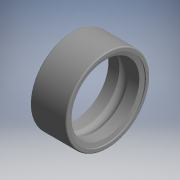
# Autodesk Inventor part: W 638/3-2Z_PART2
Saved by Autodesk Inventor 2017.3 (Build 213256000, 256)
## iProperties
Part Number: W 638/3-2Z_PART2
Material: Generic
Catalog Web Link: www.cadenas.de
Description: -Deep groove ball bearings
Vendor: SKF
Document SubType Name: Modeling
Designer: partserver
Manufacturer: SKF
Mass: 0.0355335 g
Surface Area: 1.47761 cm^2
Volume: 0.0355335 cm^3
Density: 1 g/cm^3
Appearance: PSOLRGB-175-175-175
Category: PARTsolutions
Company: SKF
Title: W 638/3-2Z_PART2
Author: Cadenas PARTsolutions
Comments: Deep groove ball bearings
PSOL_IDENT_0: {$CADENAS_DATA\23d-libs\skf_r32\bearings_units_and_housings\ball_bearings\deep_groove_ball_bearings\
PSOL_IDENT_1: bb1_001_101.prj},199 {VTYP=3D},{NB=W 638/3-2Z_PART2},{LINA=W 638/3-2Z_PART2},{NN=BB1_001_101_PART2},
PSOL_IDENT_2: {NOPRJ=TRUE},{DATE=03.04.2020 14:22:31},{GEOMDATE=30.03.2020 16:10:03},{VERSION=},{LINEID=19220},{WB
PSOL_IDENT_3: VAR=},{WBNUMERIC=}  {NB=W 638/3-2Z_PART2},{LINA=W 638/3-2Z_PART2},{KT=DUMMY},{DESIGNATION=W 638/3-2Z
PSOL_IDENT_4: },{DD=3.000},{D=7.000},{B=3.000},{C=0.000},{DD1=0.00},{DD2=3.90},{D1=0.00},{D2=6.35},{D3=0.000},{D4=
PSOL_IDENT_5: 0.000},{HH=MIN},{BB=0.000},{FF=0.00},{R0MAX=MIN},{R0=MIN},{R12=0.10},{PITCH=5.00},{DW=1.000},{DDAMIN=
PSOL_IDENT_6: 3.700},{DDAMAX=3.800},{DDBMIN=MIN},{DDBMAX=MIN},{DBMIN=MIN},{DAMAX=6.500},{BBAMIN=MIN},{CAMAX=MIN},{
PSOL_IDENT_7: RAMAX=0.100},{LOAD1=0.178},{LOAD2=0.057},{LOAD3=0.002},{SPEED1=160000},{SPEED2=80000},{KR=0.020},{F0=
PSOL_IDENT_8: 7.100},{Z=8},{II=1},{MASS=0.000},{BEARING=W 638/3-2Z},{RING=},{HELP=0.665},{HELP2=0.325},{DD1ALG=2.0
PSOL_IDENT_9: 00},{YALG=2.175},{PITCH1=5.000},{DW1=1.000},{YALG1=2.835},{HALG1=0.665},{SH=1.950},{CU=0.400},{DESIG
PSOL_IDENT_10: N=dgbbw2z},{HALG=0.675},{B1=0},{SHIELDHELP=2}
NB: W 638/3-2Z_PART2
NT: Deep groove ball bearings
NBSYN: $DESIGNATION._PART2
LINA: W 638/3-2Z_PART2
CATALOG: SKF
SUPPLIER: SKF
ARTICLENO: W 638/3-2Z_PART2
BOMINFO: W 638/3-2Z_PART2
CREATOR: CADENAS GmbH
Autodesk Inventor part; units mm, degrees
ref_plane "YZ Plane" through (0, 0, 0) normal (1, 0, 0) x (0, 1, 0)
ref_plane "XZ Plane" through (0, 0, 0) normal (0, 1, 0) x (-1, 0, 0)
ref_plane "XY Plane" through (0, 0, 0) normal (0, 0, 1) x (1, 0, 0)
sketch "Sketch_17" plane through (0, 0, 0) normal (0, 0, 1) x (1, 0, 0)
  line L0 (50, 0) -> (-50, 0)
  line L1 (0, 3.4) -> (0, 3.175)
  line L2 (0, 3.175) -> (0.03, 3.175)
  arc A0 (0.15, 3.175) -> (0.03, 3.175) centre (0.09, 3.175) ccw
  line L3 (0.15, 3.175) -> (0.21, 2.835)
  line L4 (0.21, 2.835) -> (1.1288, 2.835)
  arc A1 (1.8712, 2.835) -> (1.1288, 2.835) centre (1.5, 2.5) ccw
  line L5 (1.8712, 2.835) -> (2.79, 2.835)
  line L6 (2.79, 2.835) -> (2.85, 3.175)
  arc A2 (2.97, 3.175) -> (2.85, 3.175) centre (2.91, 3.175) ccw
  line L7 (2.97, 3.175) -> (3, 3.175)
  line L8 (3, 3.175) -> (3, 3.4)
  arc A3 (3, 3.4) -> (2.9, 3.5) centre (2.9, 3.4) ccw
  line L9 (2.9, 3.5) -> (0.1, 3.5)
  arc A4 (0.1, 3.5) -> (0, 3.4) centre (0.1, 3.4) ccw
  constraints: 20 end point, 10 point on circle, 5 centre point
revolve "Revolution1" add sketch "Sketch_17" angle 360 about axis through (50, 0, 0) along (1, 0, 0)
body "Solid1"
